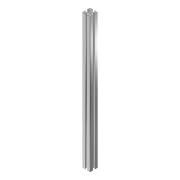
# Autodesk Inventor part: Propile_600
Saved by Autodesk Inventor 2019 (Build 230136000, 136)
## iProperties
Created: 2019-04-24
Part Number: Propile_600
Material: 알루미늄 6061
Document SubType Name: Modeling
Designer: hinmo
Density: 2.7 g/cm^3
Appearance: 알루미늄 - 평지
Mass: 520.574 g
Surface Area: 2225.94 cm^2
Volume: 192.805 cm^3
Author: hinmo
Autodesk Inventor part; units mm, degrees
ref_plane "YZ Plane" through (0, 0, 0) normal (1, 0, 0) x (0, 1, 0)
ref_plane "XZ Plane" through (0, 0, 0) normal (0, 1, 0) x (-1, 0, 0)
ref_plane "XY Plane" through (0, 0, 0) normal (0, 0, 1) x (1, 0, 0)
sketch "스케치1" plane through (0, 0, 0) normal (0, 1, 0) x (-1, 0, 0)
  arc A0 (-211.6172, 3.4366) -> (-210.6172, 4.4366) centre (-211.6172, 4.4366) ccw projected
  line L0 (-210.6172, 4.4366) -> (-210.6172, 5.9366) projected
  line L1 (-210.6172, 5.9366) -> (-212.5672, 5.9366) projected
  line L2 (-212.5672, 5.9366) -> (-213.5459, 9.6298) projected
  arc A1 (-210.9022, 13.9366) -> (-213.5459, 9.6298) centre (-206.87, 8.4967) ccw projected
  line L3 (-210.9022, 13.9366) -> (-207.9672, 13.9366) projected
  line L4 (-207.9672, 13.9366) -> (-207.4672, 14.4366) projected
  line L5 (-207.4672, 14.4366) -> (-206.9672, 13.9366) projected
  line L6 (-206.9672, 13.9366) -> (-204.0322, 13.9366) projected
  arc A2 (-201.3885, 9.6298) -> (-204.0322, 13.9366) centre (-208.0644, 8.4967) ccw projected
  line L7 (-201.3885, 9.6298) -> (-202.3672, 5.9366) projected
  line L8 (-202.3672, 5.9366) -> (-204.3172, 5.9366) projected
  line L9 (-204.3172, 5.9366) -> (-204.3172, 4.4366) projected
  arc A3 (-204.3172, 4.4366) -> (-203.3172, 3.4366) centre (-203.3172, 4.4366) ccw projected
  line L10 (-203.3172, 3.4366) -> (-193.9672, 3.4366) projected
  arc A4 (-193.9672, 3.4366) -> (-192.4672, 4.9366) centre (-193.9672, 4.9366) ccw projected
  line L11 (-192.4672, 4.9366) -> (-192.4672, 14.2866) projected
  arc A5 (-192.4672, 14.2866) -> (-193.4672, 15.2866) centre (-193.4672, 14.2866) ccw projected
  line L12 (-193.4672, 15.2866) -> (-194.9672, 15.2866) projected
  line L13 (-194.9672, 15.2866) -> (-194.9672, 13.3366) projected
  line L14 (-194.9672, 13.3366) -> (-198.6603, 12.3579) projected
  arc A6 (-202.9672, 15.0016) -> (-198.6603, 12.3579) centre (-197.5272, 19.0338) ccw projected
  line L15 (-202.9672, 15.0016) -> (-202.9672, 17.9366) projected
  line L16 (-202.9672, 17.9366) -> (-203.4672, 18.4366) projected
  line L17 (-203.4672, 18.4366) -> (-202.9672, 18.9366) projected
  line L18 (-202.9672, 18.9366) -> (-202.9672, 21.8716) projected
  arc A7 (-198.6603, 24.5154) -> (-202.9672, 21.8716) centre (-197.5272, 17.8394) ccw projected
  line L19 (-198.6603, 24.5154) -> (-194.9672, 23.5366) projected
  line L20 (-194.9672, 23.5366) -> (-194.9672, 21.5866) projected
  line L21 (-194.9672, 21.5866) -> (-193.4672, 21.5866) projected
  arc A8 (-193.4672, 21.5866) -> (-192.4672, 22.5866) centre (-193.4672, 22.5866) ccw projected
  line L22 (-192.4672, 22.5866) -> (-192.4672, 31.9366) projected
  arc A9 (-192.4672, 31.9366) -> (-193.9672, 33.4366) centre (-193.9672, 31.9366) ccw projected
  line L23 (-193.9672, 33.4366) -> (-203.3172, 33.4366) projected
  arc A10 (-203.3172, 33.4366) -> (-204.3172, 32.4366) centre (-203.3172, 32.4366) ccw projected
  line L24 (-204.3172, 32.4366) -> (-204.3172, 30.9366) projected
  line L25 (-204.3172, 30.9366) -> (-202.3672, 30.9366) projected
  line L26 (-202.3672, 30.9366) -> (-201.3885, 27.2435) projected
  arc A11 (-204.0322, 22.9366) -> (-201.3885, 27.2435) centre (-208.0644, 28.3766) ccw projected
  line L27 (-204.0322, 22.9366) -> (-206.9672, 22.9366) projected
  line L28 (-206.9672, 22.9366) -> (-207.4672, 22.4366) projected
  line L29 (-207.4672, 22.4366) -> (-207.9672, 22.9366) projected
  line L30 (-207.9672, 22.9366) -> (-210.9022, 22.9366) projected
  arc A12 (-213.5459, 27.2435) -> (-210.9022, 22.9366) centre (-206.87, 28.3766) ccw projected
  line L31 (-213.5459, 27.2435) -> (-212.5672, 30.9366) projected
  line L32 (-212.5672, 30.9366) -> (-210.6172, 30.9366) projected
  line L33 (-210.6172, 30.9366) -> (-210.6172, 32.4366) projected
  arc A13 (-210.6172, 32.4366) -> (-211.6172, 33.4366) centre (-211.6172, 32.4366) ccw projected
  line L34 (-211.6172, 33.4366) -> (-220.9672, 33.4366) projected
  arc A14 (-220.9672, 33.4366) -> (-222.4672, 31.9366) centre (-220.9672, 31.9366) ccw projected
  line L35 (-222.4672, 31.9366) -> (-222.4672, 22.5866) projected
  arc A15 (-222.4672, 22.5866) -> (-221.4672, 21.5866) centre (-221.4672, 22.5866) ccw projected
  line L36 (-221.4672, 21.5866) -> (-219.9672, 21.5866) projected
  line L37 (-219.9672, 21.5866) -> (-219.9672, 23.5366) projected
  line L38 (-219.9672, 23.5366) -> (-216.274, 24.5154) projected
  arc A16 (-211.9672, 21.8716) -> (-216.274, 24.5154) centre (-217.4071, 17.8394) ccw projected
  line L39 (-211.9672, 21.8716) -> (-211.9672, 18.9366) projected
  line L40 (-211.9672, 18.9366) -> (-211.4672, 18.4366) projected
  line L41 (-211.4672, 18.4366) -> (-211.9672, 17.9366) projected
  line L42 (-211.9672, 17.9366) -> (-211.9672, 15.0016) projected
  arc A17 (-216.274, 12.3579) -> (-211.9672, 15.0016) centre (-217.4071, 19.0338) ccw projected
  line L43 (-216.274, 12.3579) -> (-219.9672, 13.3366) projected
  line L44 (-219.9672, 13.3366) -> (-219.9672, 15.2866) projected
  line L45 (-219.9672, 15.2866) -> (-221.4672, 15.2866) projected
  arc A18 (-221.4672, 15.2866) -> (-222.4672, 14.2866) centre (-221.4672, 14.2866) ccw projected
  line L46 (-222.4672, 14.2866) -> (-222.4672, 4.9366) projected
  arc A19 (-222.4672, 4.9366) -> (-220.9672, 3.4366) centre (-220.9672, 4.9366) ccw projected
  line L47 (-220.9672, 3.4366) -> (-211.6172, 3.4366) projected
  arc A20 (-194.8829, 26.913) -> (-194.8829, 29.9603) centre (-197.4672, 28.4366) ccw projected
  line L48 (-194.8829, 26.913) -> (-193.9368, 25.967) projected
  line L49 (-193.9368, 25.967) -> (-194.9975, 24.9063) projected
  line L50 (-194.9975, 24.9063) -> (-195.9435, 25.8524) projected
  arc A21 (-198.9908, 25.8524) -> (-195.9435, 25.8524) centre (-197.4672, 28.4366) ccw projected
  line L51 (-198.9908, 25.8524) -> (-199.9368, 24.9063) projected
  line L52 (-199.9368, 24.9063) -> (-200.9975, 25.967) projected
  line L53 (-200.9975, 25.967) -> (-200.0515, 26.913) projected
  arc A22 (-200.0515, 29.9603) -> (-200.0515, 26.913) centre (-197.4672, 28.4366) ccw projected
  line L54 (-200.0515, 29.9603) -> (-200.9975, 30.9063) projected
  line L55 (-200.9975, 30.9063) -> (-199.9368, 31.967) projected
  line L56 (-199.9368, 31.967) -> (-198.9908, 31.0209) projected
  arc A23 (-195.9435, 31.0209) -> (-198.9908, 31.0209) centre (-197.4672, 28.4366) ccw projected
  line L57 (-195.9435, 31.0209) -> (-194.9975, 31.967) projected
  line L58 (-194.9975, 31.967) -> (-193.9368, 30.9063) projected
  line L59 (-193.9368, 30.9063) -> (-194.8829, 29.9603) projected
  line L60 (-204.4368, 20.4063) -> (-205.371, 19.7991) projected
  arc A24 (-205.371, 17.0742) -> (-205.371, 19.7991) centre (-207.4672, 18.4366) ccw projected
  line L61 (-205.371, 17.0742) -> (-204.4368, 16.467) projected
  line L62 (-204.4368, 16.467) -> (-205.4975, 15.4063) projected
  line L63 (-205.4975, 15.4063) -> (-206.1047, 16.3405) projected
  arc A25 (-208.8296, 16.3405) -> (-206.1047, 16.3405) centre (-207.4672, 18.4366) ccw projected
  line L64 (-208.8296, 16.3405) -> (-209.4368, 15.4063) projected
  line L65 (-209.4368, 15.4063) -> (-210.4975, 16.467) projected
  line L66 (-210.4975, 16.467) -> (-209.5633, 17.0742) projected
  arc A26 (-209.5633, 19.7991) -> (-209.5633, 17.0742) centre (-207.4672, 18.4366) ccw projected
  line L67 (-209.5633, 19.7991) -> (-210.4975, 20.4063) projected
  line L68 (-210.4975, 20.4063) -> (-209.4368, 21.467) projected
  line L69 (-209.4368, 21.467) -> (-208.8296, 20.5328) projected
  arc A27 (-206.1047, 20.5328) -> (-208.8296, 20.5328) centre (-207.4672, 18.4366) ccw projected
  line L70 (-206.1047, 20.5328) -> (-205.4975, 21.467) projected
  line L71 (-205.4975, 21.467) -> (-204.4368, 20.4063) projected
  arc A28 (-195.9435, 11.0209) -> (-198.9908, 11.0209) centre (-197.4672, 8.4366) ccw projected
  line L72 (-195.9435, 11.0209) -> (-194.9975, 11.967) projected
  line L73 (-194.9975, 11.967) -> (-193.9368, 10.9063) projected
  line L74 (-193.9368, 10.9063) -> (-194.8829, 9.9603) projected
  arc A29 (-194.8829, 6.913) -> (-194.8829, 9.9603) centre (-197.4672, 8.4366) ccw projected
  line L75 (-194.8829, 6.913) -> (-193.9368, 5.967) projected
  line L76 (-193.9368, 5.967) -> (-194.9975, 4.9063) projected
  line L77 (-194.9975, 4.9063) -> (-195.9435, 5.8524) projected
  arc A30 (-198.9908, 5.8524) -> (-195.9435, 5.8524) centre (-197.4672, 8.4366) ccw projected
  line L78 (-198.9908, 5.8524) -> (-199.9368, 4.9063) projected
  line L79 (-199.9368, 4.9063) -> (-200.9975, 5.967) projected
  line L80 (-200.9975, 5.967) -> (-200.0515, 6.913) projected
  arc A31 (-200.0515, 9.9603) -> (-200.0515, 6.913) centre (-197.4672, 8.4366) ccw projected
  line L81 (-200.0515, 9.9603) -> (-200.9975, 10.9063) projected
  line L82 (-200.9975, 10.9063) -> (-199.9368, 11.967) projected
  line L83 (-199.9368, 11.967) -> (-198.9908, 11.0209) projected
  arc A32 (-218.9908, 25.8524) -> (-215.9435, 25.8524) centre (-217.4672, 28.4366) ccw projected
  line L84 (-218.9908, 25.8524) -> (-219.9368, 24.9063) projected
  line L85 (-219.9368, 24.9063) -> (-220.9975, 25.967) projected
  line L86 (-220.9975, 25.967) -> (-220.0515, 26.913) projected
  arc A33 (-220.0515, 29.9603) -> (-220.0515, 26.913) centre (-217.4672, 28.4366) ccw projected
  line L87 (-220.0515, 29.9603) -> (-220.9975, 30.9063) projected
  line L88 (-220.9975, 30.9063) -> (-219.9368, 31.967) projected
  line L89 (-219.9368, 31.967) -> (-218.9908, 31.0209) projected
  arc A34 (-215.9435, 31.0209) -> (-218.9908, 31.0209) centre (-217.4672, 28.4366) ccw projected
  line L90 (-215.9435, 31.0209) -> (-214.9975, 31.967) projected
  line L91 (-214.9975, 31.967) -> (-213.9368, 30.9063) projected
  line L92 (-213.9368, 30.9063) -> (-214.8829, 29.9603) projected
  arc A35 (-214.8829, 26.913) -> (-214.8829, 29.9603) centre (-217.4672, 28.4366) ccw projected
  line L93 (-214.8829, 26.913) -> (-213.9368, 25.967) projected
  line L94 (-213.9368, 25.967) -> (-214.9975, 24.9063) projected
  line L95 (-214.9975, 24.9063) -> (-215.9435, 25.8524) projected
  arc A36 (-214.8829, 6.913) -> (-214.8829, 9.9603) centre (-217.4672, 8.4366) ccw projected
  line L96 (-214.8829, 6.913) -> (-213.9368, 5.967) projected
  line L97 (-213.9368, 5.967) -> (-214.9975, 4.9063) projected
  line L98 (-214.9975, 4.9063) -> (-215.9435, 5.8524) projected
  arc A37 (-218.9908, 5.8524) -> (-215.9435, 5.8524) centre (-217.4672, 8.4366) ccw projected
  line L99 (-218.9908, 5.8524) -> (-219.9368, 4.9063) projected
  line L100 (-219.9368, 4.9063) -> (-220.9975, 5.967) projected
  line L101 (-220.9975, 5.967) -> (-220.0515, 6.913) projected
  arc A38 (-220.0515, 9.9603) -> (-220.0515, 6.913) centre (-217.4672, 8.4366) ccw projected
  line L102 (-220.0515, 9.9603) -> (-220.9975, 10.9063) projected
  line L103 (-220.9975, 10.9063) -> (-219.9368, 11.967) projected
  line L104 (-219.9368, 11.967) -> (-218.9908, 11.0209) projected
  arc A39 (-215.9435, 11.0209) -> (-218.9908, 11.0209) centre (-217.4672, 8.4366) ccw projected
  line L105 (-215.9435, 11.0209) -> (-214.9975, 11.967) projected
  line L106 (-214.9975, 11.967) -> (-213.9368, 10.9063) projected
  line L107 (-213.9368, 10.9063) -> (-214.8829, 9.9603) projected
  arc A40 (-4.15, -15) -> (-3.15, -14) centre (-4.15, -14) ccw
  line L108 (-3.15, -14) -> (-3.15, -12.5)
  line L109 (-3.15, -12.5) -> (-5.1, -12.5)
  line L110 (-5.1, -12.5) -> (-6.0787, -8.8068)
  arc A41 (-3.435, -4.5) -> (-6.0787, -8.8068) centre (0.5972, -9.94) ccw
  line L111 (-3.435, -4.5) -> (-0.5, -4.5)
  line L112 (-0.5, -4.5) -> (0, -4)
  line L113 (0, -4) -> (0.5, -4.5)
  line L114 (0.5, -4.5) -> (3.435, -4.5)
  arc A42 (6.0787, -8.8068) -> (3.435, -4.5) centre (-0.5972, -9.94) ccw
  line L115 (6.0787, -8.8068) -> (5.1, -12.5)
  line L116 (5.1, -12.5) -> (3.15, -12.5)
  line L117 (3.15, -12.5) -> (3.15, -14)
  arc A43 (3.15, -14) -> (4.15, -15) centre (4.15, -14) ccw
  line L118 (4.15, -15) -> (13.5, -15)
  arc A44 (13.5, -15) -> (15, -13.5) centre (13.5, -13.5) ccw
  line L119 (15, -13.5) -> (15, -4.15)
  arc A45 (15, -4.15) -> (14, -3.15) centre (14, -4.15) ccw
  line L120 (14, -3.15) -> (12.5, -3.15)
  line L121 (12.5, -3.15) -> (12.5, -5.1)
  line L122 (12.5, -5.1) -> (8.8068, -6.0787)
  arc A46 (4.5, -3.435) -> (8.8068, -6.0787) centre (9.94, 0.5972) ccw
  line L123 (4.5, -3.435) -> (4.5, -0.5)
  line L124 (4.5, -0.5) -> (4, 0)
  line L125 (4, 0) -> (4.5, 0.5)
  line L126 (4.5, 0.5) -> (4.5, 3.435)
  arc A47 (8.8068, 6.0787) -> (4.5, 3.435) centre (9.94, -0.5972) ccw
  line L127 (8.8068, 6.0787) -> (12.5, 5.1)
  line L128 (12.5, 5.1) -> (12.5, 3.15)
  line L129 (12.5, 3.15) -> (14, 3.15)
  arc A48 (14, 3.15) -> (15, 4.15) centre (14, 4.15) ccw
  line L130 (15, 4.15) -> (15, 13.5)
  arc A49 (15, 13.5) -> (13.5, 15) centre (13.5, 13.5) ccw
  line L131 (13.5, 15) -> (4.15, 15)
  arc A50 (4.15, 15) -> (3.15, 14) centre (4.15, 14) ccw
  line L132 (3.15, 14) -> (3.15, 12.5)
  line L133 (3.15, 12.5) -> (5.1, 12.5)
  line L134 (5.1, 12.5) -> (6.0787, 8.8068)
  arc A51 (3.435, 4.5) -> (6.0787, 8.8068) centre (-0.5972, 9.94) ccw
  line L135 (3.435, 4.5) -> (0.5, 4.5)
  line L136 (0.5, 4.5) -> (0, 4)
  line L137 (0, 4) -> (-0.5, 4.5)
  line L138 (-0.5, 4.5) -> (-3.435, 4.5)
  arc A52 (-6.0787, 8.8068) -> (-3.435, 4.5) centre (0.5972, 9.94) ccw
  line L139 (-6.0787, 8.8068) -> (-5.1, 12.5)
  line L140 (-5.1, 12.5) -> (-3.15, 12.5)
  line L141 (-3.15, 12.5) -> (-3.15, 14)
  arc A53 (-3.15, 14) -> (-4.15, 15) centre (-4.15, 14) ccw
  line L142 (-4.15, 15) -> (-13.5, 15)
  arc A54 (-13.5, 15) -> (-15, 13.5) centre (-13.5, 13.5) ccw
  line L143 (-15, 13.5) -> (-15, 4.15)
  arc A55 (-15, 4.15) -> (-14, 3.15) centre (-14, 4.15) ccw
  line L144 (-14, 3.15) -> (-12.5, 3.15)
  line L145 (-12.5, 3.15) -> (-12.5, 5.1)
  line L146 (-12.5, 5.1) -> (-8.8068, 6.0787)
  arc A56 (-4.5, 3.435) -> (-8.8068, 6.0787) centre (-9.94, -0.5972) ccw
  line L147 (-4.5, 3.435) -> (-4.5, 0.5)
  line L148 (-4.5, 0.5) -> (-4, 0)
  line L149 (-4, 0) -> (-4.5, -0.5)
  line L150 (-4.5, -0.5) -> (-4.5, -3.435)
  arc A57 (-8.8068, -6.0787) -> (-4.5, -3.435) centre (-9.94, 0.5972) ccw
  line L151 (-8.8068, -6.0787) -> (-12.5, -5.1)
  line L152 (-12.5, -5.1) -> (-12.5, -3.15)
  line L153 (-12.5, -3.15) -> (-14, -3.15)
  arc A58 (-14, -3.15) -> (-15, -4.15) centre (-14, -4.15) ccw
  line L154 (-15, -4.15) -> (-15, -13.5)
  arc A59 (-15, -13.5) -> (-13.5, -15) centre (-13.5, -13.5) ccw
  line L155 (-13.5, -15) -> (-4.15, -15)
  arc A60 (12.5843, 8.4764) -> (12.5843, 11.5236) centre (10, 10) ccw
  line L156 (12.5843, 8.4764) -> (13.5303, 7.5303)
  line L157 (13.5303, 7.5303) -> (12.4697, 6.4697)
  line L158 (12.4697, 6.4697) -> (11.5236, 7.4157)
  arc A61 (8.4764, 7.4157) -> (11.5236, 7.4157) centre (10, 10) ccw
  line L159 (8.4764, 7.4157) -> (7.5303, 6.4697)
  line L160 (7.5303, 6.4697) -> (6.4697, 7.5303)
  line L161 (6.4697, 7.5303) -> (7.4157, 8.4764)
  arc A62 (7.4157, 11.5236) -> (7.4157, 8.4764) centre (10, 10) ccw
  line L162 (7.4157, 11.5236) -> (6.4697, 12.4697)
  line L163 (6.4697, 12.4697) -> (7.5303, 13.5303)
  line L164 (7.5303, 13.5303) -> (8.4764, 12.5843)
  arc A63 (11.5236, 12.5843) -> (8.4764, 12.5843) centre (10, 10) ccw
  line L165 (11.5236, 12.5843) -> (12.4697, 13.5303)
  line L166 (12.4697, 13.5303) -> (13.5303, 12.4697)
  line L167 (13.5303, 12.4697) -> (12.5843, 11.5236)
  line L168 (3.0303, 1.9697) -> (2.0961, 1.3624)
  arc A64 (2.0961, -1.3624) -> (2.0961, 1.3624) centre (0, 0) ccw
  line L169 (2.0961, -1.3624) -> (3.0303, -1.9697)
  line L170 (3.0303, -1.9697) -> (1.9697, -3.0303)
  line L171 (1.9697, -3.0303) -> (1.3624, -2.0961)
  arc A65 (-1.3624, -2.0961) -> (1.3624, -2.0961) centre (0, 0) ccw
  line L172 (-1.3624, -2.0961) -> (-1.9697, -3.0303)
  line L173 (-1.9697, -3.0303) -> (-3.0303, -1.9697)
  line L174 (-3.0303, -1.9697) -> (-2.0961, -1.3624)
  arc A66 (-2.0961, 1.3624) -> (-2.0961, -1.3624) centre (0, 0) ccw
  line L175 (-2.0961, 1.3624) -> (-3.0303, 1.9697)
  line L176 (-3.0303, 1.9697) -> (-1.9697, 3.0303)
  line L177 (-1.9697, 3.0303) -> (-1.3624, 2.0961)
  arc A67 (1.3624, 2.0961) -> (-1.3624, 2.0961) centre (0, 0) ccw
  line L178 (1.3624, 2.0961) -> (1.9697, 3.0303)
  line L179 (1.9697, 3.0303) -> (3.0303, 1.9697)
  arc A68 (11.5236, -7.4157) -> (8.4764, -7.4157) centre (10, -10) ccw
  line L180 (11.5236, -7.4157) -> (12.4697, -6.4697)
  line L181 (12.4697, -6.4697) -> (13.5303, -7.5303)
  line L182 (13.5303, -7.5303) -> (12.5843, -8.4764)
  arc A69 (12.5843, -11.5236) -> (12.5843, -8.4764) centre (10, -10) ccw
  line L183 (12.5843, -11.5236) -> (13.5303, -12.4697)
  line L184 (13.5303, -12.4697) -> (12.4697, -13.5303)
  line L185 (12.4697, -13.5303) -> (11.5236, -12.5843)
  arc A70 (8.4764, -12.5843) -> (11.5236, -12.5843) centre (10, -10) ccw
  line L186 (8.4764, -12.5843) -> (7.5303, -13.5303)
  line L187 (7.5303, -13.5303) -> (6.4697, -12.4697)
  line L188 (6.4697, -12.4697) -> (7.4157, -11.5236)
  arc A71 (7.4157, -8.4764) -> (7.4157, -11.5236) centre (10, -10) ccw
  line L189 (7.4157, -8.4764) -> (6.4697, -7.5303)
  line L190 (6.4697, -7.5303) -> (7.5303, -6.4697)
  line L191 (7.5303, -6.4697) -> (8.4764, -7.4157)
  arc A72 (-11.5236, 7.4157) -> (-8.4764, 7.4157) centre (-10, 10) ccw
  line L192 (-11.5236, 7.4157) -> (-12.4697, 6.4697)
  line L193 (-12.4697, 6.4697) -> (-13.5303, 7.5303)
  line L194 (-13.5303, 7.5303) -> (-12.5843, 8.4764)
  arc A73 (-12.5843, 11.5236) -> (-12.5843, 8.4764) centre (-10, 10) ccw
  line L195 (-12.5843, 11.5236) -> (-13.5303, 12.4697)
  line L196 (-13.5303, 12.4697) -> (-12.4697, 13.5303)
  line L197 (-12.4697, 13.5303) -> (-11.5236, 12.5843)
  arc A74 (-8.4764, 12.5843) -> (-11.5236, 12.5843) centre (-10, 10) ccw
  line L198 (-8.4764, 12.5843) -> (-7.5303, 13.5303)
  line L199 (-7.5303, 13.5303) -> (-6.4697, 12.4697)
  line L200 (-6.4697, 12.4697) -> (-7.4157, 11.5236)
  arc A75 (-7.4157, 8.4764) -> (-7.4157, 11.5236) centre (-10, 10) ccw
  line L201 (-7.4157, 8.4764) -> (-6.4697, 7.5303)
  line L202 (-6.4697, 7.5303) -> (-7.5303, 6.4697)
  line L203 (-7.5303, 6.4697) -> (-8.4764, 7.4157)
  arc A76 (-7.4157, -11.5236) -> (-7.4157, -8.4764) centre (-10, -10) ccw
  line L204 (-7.4157, -11.5236) -> (-6.4697, -12.4697)
  line L205 (-6.4697, -12.4697) -> (-7.5303, -13.5303)
  line L206 (-7.5303, -13.5303) -> (-8.4764, -12.5843)
  arc A77 (-11.5236, -12.5843) -> (-8.4764, -12.5843) centre (-10, -10) ccw
  line L207 (-11.5236, -12.5843) -> (-12.4697, -13.5303)
  line L208 (-12.4697, -13.5303) -> (-13.5303, -12.4697)
  line L209 (-13.5303, -12.4697) -> (-12.5843, -11.5236)
  arc A78 (-12.5843, -8.4764) -> (-12.5843, -11.5236) centre (-10, -10) ccw
  line L210 (-12.5843, -8.4764) -> (-13.5303, -7.5303)
  line L211 (-13.5303, -7.5303) -> (-12.4697, -6.4697)
  line L212 (-12.4697, -6.4697) -> (-11.5236, -7.4157)
  arc A79 (-8.4764, -7.4157) -> (-11.5236, -7.4157) centre (-10, -10) ccw
  line L213 (-8.4764, -7.4157) -> (-7.5303, -6.4697)
  line L214 (-7.5303, -6.4697) -> (-6.4697, -7.5303)
  line L215 (-6.4697, -7.5303) -> (-7.4157, -8.4764)
  point P0 (0, 0)
  constraints: 216 end point, 80 point on circle, 40 centre point
extrude "돌출1" add sketch "스케치1" along normal blind 500 contours L155 A59 L154 A58 L153 L152 L151 A57 L150 L149 L148 L147 A56 L146 L145 L144 A55 L143 A54 L142 A53 L141 L140 L139 A52 L138 L137 L136 L135 A51 L134 L133 L132 A50 L131 A49 L130 A48 L129 L128 L127 A47 L126 L125 L124 L123 A46 L122 L121 L120 A45 L119 A44 L118 A43 L117 L116 L115 A42 L114 L113 L112 L111 A41 L110 L109 L108 A40
